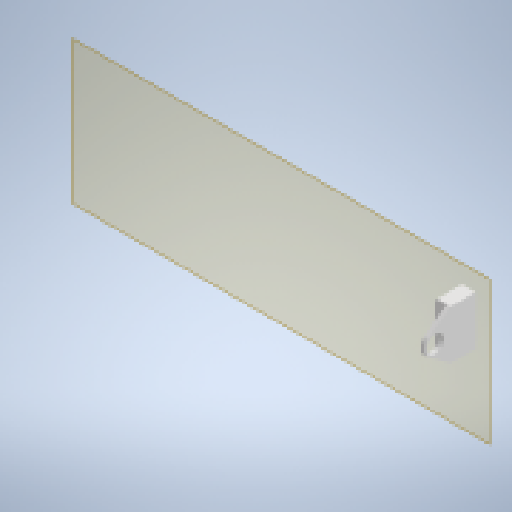
# Autodesk Inventor part: tumbler_holdeerr
Saved by Autodesk Inventor 2024 (Build 280153000, 153)
## iProperties
Created: 2026-03-14
Part Number: tumbler_holdeerr
Material: Generic
Document SubType Name: Modeling
Designer: SEMEN
Density: 1 g/cm^3
Appearance: Default
Author: SEMEN
Autodesk Inventor part; units mm, degrees
ref_plane "YZ Plane" through (0, 0, 0) normal (1, 0, 0) x (0, 1, 0)
ref_plane "XZ Plane" through (0, 0, 0) normal (0, 1, 0) x (-1, 0, 0)
ref_plane "Work Plane1" through (0, 0, 0) normal (0, 0, 1) x (1, 0, 0)
sketch "Sketch1" plane through (0, 0, 0) normal (0, 0, 1) x (1, 0, 0)
  circle A0 centre (119.5, 7) radius 3.3 projected
  circle A1 centre (119.5, 38) radius 3.3 projected
  circle A2 centre (88.5, 38) radius 3.3 projected
  circle A3 centre (88.5, 7) radius 3.3 projected
  circle A4 centre (104, 22.5) radius 11 projected
  circle A5 centre (-76, 8.5) radius 1.7 projected
  circle A6 centre (-76, 38) radius 1.7 projected
  circle A7 centre (-45, -33.5) radius 4.3 projected
  circle A8 centre (-45, -3) radius 4.3 projected
  circle A9 centre (-60.5, 12.5) radius 1.7 projected
  circle A10 centre (-60.5, 43.5) radius 1.7 projected
  circle A11 centre (-29.5, 43.5) radius 1.7 projected
  circle A12 centre (-29.5, 12.5) radius 1.7 projected
  circle A13 centre (-45, 28) radius 11.5 projected
  circle A14 centre (-122.5, -32.5) radius 3.3 projected
  circle A15 centre (-83.5, -32.5) radius 3.3 projected
  circle A16 centre (83.5, -32.5) radius 3.3 projected
  circle A17 centre (122.5, -32.5) radius 3.3 projected
  circle A18 centre (-103, 22.5) radius 2.75 projected
  circle A19 centre (78, 8.5) radius 1.7 projected
  circle A20 centre (78, 38) radius 1.7 projected
  circle A21 centre (-130, 8.5) radius 1.7 projected
  circle A22 centre (-130, 38) radius 1.7 projected
  circle A23 centre (130, 38) radius 1.7 projected
  circle A24 centre (130, 8.5) radius 1.7 projected
  arc A25 (-135, -38.5) -> (-130, -43.5) centre (-130, -38.5) ccw projected
  line L0 (130, -43.5) -> (-130, -43.5) projected
  arc A26 (130, -43.5) -> (135, -38.5) centre (130, -38.5) ccw projected
  line L1 (135, 38.5) -> (135, -38.5) projected
  arc A27 (135, 38.5) -> (130, 43.5) centre (130, 38.5) ccw projected
  line L2 (-24, 43.5) -> (130, 43.5) projected
  line L3 (-24, 43.5) -> (-24, 45.5) projected
  line L4 (-24, 45.5) -> (-27.5, 49) projected
  line L5 (-27.5, 49) -> (-62.5, 49) projected
  line L6 (-62.5, 49) -> (-66, 45.5) projected
  line L7 (-66, 45.5) -> (-66, 43.5) projected
  line L8 (-130, 43.5) -> (-66, 43.5) projected
  arc A28 (-130, 43.5) -> (-135, 38.5) centre (-130, 38.5) ccw projected
  line L9 (-135, -38.5) -> (-135, 38.5) projected
  line L10 (-115.5, -26.5) -> (-115.5, -38.5) projected
  line L11 (-90.5, -26.5) -> (-115.5, -26.5) projected
  line L12 (-90.5, -38.5) -> (-90.5, -26.5) projected
  line L13 (-115.5, -38.5) -> (-90.5, -38.5) projected
  line L14 (117.5, -38.5) -> (117.5, -26.5) projected
  line L15 (90.5, -38.5) -> (117.5, -38.5) projected
  line L16 (90.5, -26.5) -> (90.5, -38.5) projected
  line L17 (117.5, -26.5) -> (90.5, -26.5) projected
  line L18 (130, 38) -> (130, 8.5) construction
  line L19 (127.3, 38) -> (127.3, 8.5)
  arc A29 (130, 40.7) -> (127.3, 38) centre (130, 38) ccw
  arc A30 (127.3, 8.5) -> (130, 5.8) centre (130, 8.5) ccw
  line L20 (135, 38.5) -> (135, 40.7)
  line L21 (130, 5.8) -> (138.5, 5.8)
  line L22 (135.5, 40.7) -> (135.5, 5.8)
  line L23 (138.5, 40.7) -> (138.5, 5.8)
  line L24 (138.5, 40.7) -> (130, 40.7)
  point P0 (0, 0)
  point P1 (130, 23.25)
  dimension "d0" = 5.4
  dimension "d1" = 0.5
  dimension "d2" = 3
  constraints: 16 end point, 4 point on circle, 4 tangent, 4 vertical, 3 point on line, 2 centre point, 1 equal radius, 1 horizontal, 1 midpoint, 1 perpendicular
  measures "d0" diameter of A30
  measures "d1" distance between parallel lines of L20 L22
  measures "d2" distance between parallel lines of L22 L23
ref_plane "Work Plane2" through (-135, -43.5, 18) normal (0, 0, -1) x (0, 1, 0)
extrude "Extrusion1" add sketch "Sketch1" along normal up to surface (18 mm away) contours A23 | A24 | L21 A30 L19 A29 L24 A27 L1 | L1 L20 L24 L22 L21 | A27 L24 L20 | L22 L24 L23 L21
sketch "Sketch2" plane through (130, 40.7, 18) normal (0, 0, 1) x (1, 0, 0)
  arc A0 (0, 0) -> (-2.7, -2.7) centre (0, -2.7) ccw projected
  line L0 (8.5, 0) -> (0, 0) projected
  line L1 (8.5, -34.9) -> (8.5, 0) projected
  line L2 (0, -34.9) -> (8.5, -34.9) projected
  arc A1 (-2.7, -32.2) -> (0, -34.9) centre (0, -32.2) ccw projected
  line L3 (-2.7, -2.7) -> (-2.7, -32.2) projected
  line L4 (5.5, 0) -> (5.5, -34.9) projected
  line L5 (5, -2.2) -> (5, 0) projected
  line L6 (5, -2.2) -> (5, -79.2) projected
  point P0 (-130, -40.7)
extrude "Extrusion2" add sketch "Sketch2" along normal blind 18 contours L0 L1 L2 L4
sketch "Sketch3" plane through (138.5, 5.8, 0) normal (1, 0, 0) x (0, 0, -1)
  line L0 (-36, 0) -> (-36, 34.9) projected
  line L1 (-22, 32.7) -> (-22, -44.3) projected
  line L2 (-22, 32.7) -> (-22, 37.7) projected
  circle A0 centre (-29, 17.45) radius 7.5
  line L3 (-36, 17.45) -> (-22, 17.45) construction
  line L4 (-18, 37.7) -> (-18, 32.7) projected
  line L5 (-18, 32.7) -> (-18, -44.3) projected
  line L6 (-18, 34.9) -> (-36, 34.9) projected
  line L7 (0, 0) -> (-36, 0) projected
  line L8 (-18, 34.9) -> (-33.4562, 23.4826)
  line L9 (-33.4562, 11.4174) -> (-18, 0)
  circle A1 centre (-29, 17.45) radius 6
  point P0 (0, -5.8)
  point P1 (-36, 20.1426)
  point P2 (-36, 14.7574)
  point P3 (-22, 20.1426)
  point P4 (-22, 14.7574)
  dimension "d7" = 15
  dimension "d8" = 12
  constraints: 6 end point, 3 midpoint, 2 centre point, 2 coincident, 2 point on circle, 2 tangent, 1 perpendicular, 1 point on line
  measures "d7" diameter of A0
  measures "d8" diameter of A1
extrude "Extrusion3" cut sketch "Sketch3" against normal through all contours L0 A0 L9 L1 L7 | A0 L0 | L1 L9 L7 | L0 L6 L2 L1 L8 A0 | L6 L8 L1 L2 | A1
body "Solid1"
